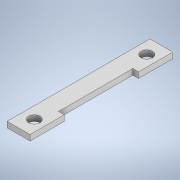
# Autodesk Inventor part: headplate_ephys
Saved by Autodesk Inventor 2022 (Build 260153000, 153)
## iProperties
Created: 2022-06-06
Part Number: headplate_ephys
Material: Generic
Document SubType Name: Modeling
Designer: Florencia
Density: 1 g/cm^3
Appearance: Default
Author: Florencia
Autodesk Inventor part; units mm, degrees
ref_plane "YZ Plane" through (0, 0, 0) normal (1, 0, 0) x (0, 1, 0)
ref_plane "XZ Plane" through (0, 0, 0) normal (0, 1, 0) x (-1, 0, 0)
ref_plane "XY Plane" through (0, 0, 0) normal (0, 0, 1) x (1, 0, 0)
sketch "Sketch1" plane through (0, 0, 0) normal (0, 1, 0) x (-1, 0, 0)
  point P0 (0, 0)
sketch "Sketch2" plane through (0, 0, 0) normal (0, 1, 0) x (-1, 0, 0)
  line L0 (0, 0) -> (4, 0)
  line L1 (4, 0) -> (4, 25)
  line L2 (4, 25) -> (0, 25)
  line L3 (0, 25) -> (0, 0)
  point P0 (3, 0)
  point P1 (0, 6)
  point P2 (0, 19)
  dimension "d0" = 4
  dimension "d1" = 25
  constraints: 8 end point, 3 point on line, 2 parallel, 1 coincident, 1 horizontal, 1 perpendicular
  measures "d0" distance of L2.end L1.end
  measures "d1" distance of L1.end L0.end
extrude "Extrusion1" add sketch "Sketch2" against normal blind 1
sketch "Sketch3" plane through (0, 0, 0) normal (0, 1, 0) x (-1, 0, 0)
  line L0 (1, 19) -> (0, 19)
  line L1 (0, 19) -> (0, 6)
  line L2 (0, 6) -> (1, 6)
  line L3 (1, 6) -> (1, 19)
  point P0 (0, 0)
  point P1 (0, 2.65)
  point P2 (0, 0)
  point P3 (0, 22.35)
  point P4 (-6.35, -25.4)
  point P5 (3, 25)
  point P6 (3, 22.35)
  point P7 (3, 2.65)
  dimension "d4" = 13
  dimension "d20" = 1
  constraints: 8 end point, 2 parallel, 1 coincident, 1 horizontal, 1 perpendicular
  measures "d4" distance of L1.end L0.end
  measures "d20" distance of L1.end L2.end
extrude "Extrusion2" cut sketch "Sketch3" against normal blind 1
sketch "Sketch6" plane through (0, 0, 0) normal (0, 1, 0) x (1, 0, 0)
  point P0 (0, 0)
sketch "Sketch7" plane through (0, 0, 0) normal (0, 1, 0) x (1, 0, 0)
  line L0 (-4, 0) -> (-4, -25) projected
  line L1 (-4, -25) -> (0, -25) projected
  point P0 (0, 0)
  point P1 (-1.9, -2.65)
  point P2 (-1.9, -22.35)
  dimension "d21" = 2.1
  dimension "d22" = 2.65
  dimension "d23" = 2.65
  dimension "d24" = 2.1
  measures "d21" distance from line of L0 point (-1.9, -2.65)
  measures "d22" vertical distance of point (0, 0) point (-1.9, -2.65)
  measures "d23" distance from line of point (-1.9, -22.35) L1
  measures "d24" horizontal distance of L0.end point (-1.9, -22.35)
hole "Hole2" at (-1.9, 0, 2.65) at (-1.9, 0, 22.35) direction (0, -1, 0) diameter 2 depth 2 tip angle 118
body "Solid1"
